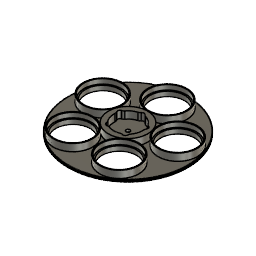
wheel_updated (Autodesk Fusion 360 design; units mm, degrees)
Autodesk Fusion 360 part; units mm, degrees
sketch "Sketch1" plane through (0, 0, 0) normal (0, 0, 1) x (1, 0, 0)
  circle A0 centre (0, 0) radius 50
  dimension "d1" = 100
  constraint coincident A0.centre origin
  measures "d1" diameter of A0
extrude "Extrude1" add sketch "Sketch1" along normal blind 2
sketch "Sketch2" plane through (0, 0, 2) normal (0, 0, 1) x (-1, 0, 0)
  circle A0 centre (0, 0) radius 50
  circle A1 centre (0, -33) radius 14.4
  circle A2 centre (0, -33) radius 16.4
  circle A3 centre (0, -33) radius 15.6
  dimension "d4" = 28.8
  dimension "d5" = 2
  dimension "d38" = 33
  dimension "d48" = 31.2
  constraint vertical A0.centre A1.centre
  constraint concentric A1 A3
  measures "d4" diameter of A1
  measures "d38" distance of A0.centre A1.centre
  measures "d48" diameter of A3
extrude "Extrude8" cut sketch "Sketch2" against normal blind 2 contours A1
extrude "Extrude9" add sketch "Sketch2" along normal blind 2 contours A3
extrude "Extrude10" add sketch "Sketch2" along normal blind 6 contours A2
pattern_circular "C-Pattern3" count 5 over 360 about axis through (0, 0, 1.75) along (0, 0, 1) of "Extrude8", "Extrude9", "Extrude10"
sketch "Sketch4" plane through (0, 0, 2) normal (0, 0, 1) x (-1, 0, 0)
  line L0 (0, 0) -> (-8.6364, -5.0411) construction
  circle A0 centre (-6.9554, 9.1582) radius 2
  circle A1 centre (-10.7716, -4.0278) radius 2
  circle A2 centre (6.9328, 9.1753) radius 2
  circle A3 centre (-0.0088, -11.5) radius 1.5 construction
  circle A4 centre (0, 0) radius 10 construction
  circle A5 centre (0, 0) radius 11.5 construction
  line L1 (0, 0) -> (8.6372, -5.0397) construction
  circle A6 centre (0, 0) radius 8.5 construction
  circle A7 centre (0, 0) radius 12
  circle A8 centre (-0.0088, -11.5) radius 2
  circle A9 centre (10.7738, -4.0219) radius 2
  circle A10 centre (0, 0) radius 50
  circle A11 centre (0, 0) radius 16.5
  circle A12 centre (0, 0) radius 1.6
  circle A13 centre (-31.3849, -10.1976) radius 16.4
  circle A14 centre (-19.3969, 26.6976) radius 16.4
  circle A15 centre (19.3969, 26.6976) radius 16.4
  circle A16 centre (31.3849, -10.1976) radius 16.4
  circle A17 centre (0, -33) radius 16.4
  point P0 (-0.0088, 0)
  dimension "d14" = 1.5
  dimension "d15" = -1.5
  dimension "d16" = 2
  dimension "d17" = 0.5
  dimension "d18" = 20
  dimension "d19" = 3
  dimension "d20" = 4
  dimension "d21" = 4
  dimension "d22" = 4
  dimension "d23" = 4
  dimension "d39" = 33
  dimension "d45" = 3.2
  constraint coincident L0.start A4.centre
  constraint coincident L1.end A4
  constraint coincident L0.end A4
  constraint coincident A3.centre A5
  constraint coincident A9.centre A5
  constraint coincident A1.centre A5
  constraint coincident A2.centre A5
  constraint coincident A0.centre A5
  constraint concentric A7 A10
  constraint concentric A10 A12
  measures "d18" diameter of A4
  measures "d19" diameter of A3
  measures "d20" diameter of A9
  measures "d21" diameter of A1
  measures "d22" diameter of A2
  measures "d23" diameter of A0
  measures "d39" diameter of A11
  measures "d45" diameter of A12
extrude "Extrude6" add sketch "Sketch4" along normal blind 6 contours A11
fillet "Fillet2" radius 3 10 edges at (-10.4, 5.9867, 5) (-11.7789, 2.2929, 5) (-1.9624, 11.8385, 5) (1.9805, 11.8354, 5) (10.3967, 5.9923, 5) (-8.7089, -8.2556, 5) (-5.5631, -10.6326, 5) (5.5893, -10.6189, 5) (8.7292, -8.2342, 5) (11.7777, 2.2993, 5)
ref_plane "WorkPlane1" through (0, -50, 0) normal (0, 1, 0) x (0, 0, 1)
sketch "Sketch5" plane through (0, -50, 0) normal (0, 1, 0) x (1, 0, 0)
  line L0 (0, 0) -> (-0.5, 0)
  line L1 (-0.5, 0) -> (-0.5, -2)
  line L2 (-0.5, -2) -> (0, -2)
  line L3 (0, -2) -> (0, 0)
  dimension "d30" = 0.5
  dimension "d31" = 2
  constraint horizontal L0
  constraint vertical L1
  constraint horizontal L2
  constraint vertical L3
  constraint coincident L0.start L3.end
  measures "d30" distance of L0.start L0.end
  measures "d31" distance of L0.start L2.end
extrude "Extrude5" cut sketch "Sketch5" along normal blind 0.25
pattern_circular "C-Pattern2" count 400 over 360 about axis through (0, 0, 1.75) along (0, 0, 1) of "Extrude5"
extrude "Extrude7" cut sketch "Sketch4" against normal blind 2 contours A12
equation "d16 = 1.50 mm + 0.5 mm"
